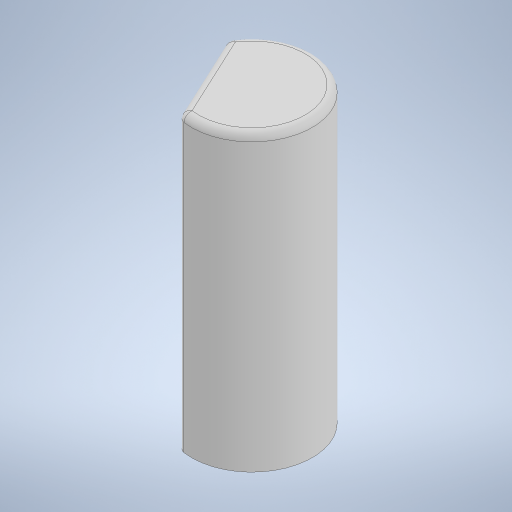
# Autodesk Inventor part: Poti_Verlaengerung
Saved by Autodesk Inventor 2023.1 (Build 271208000, 208)
## iProperties
Created: 2023-12-21
Part Number: Poti_Verlaengerung
Material: Generisch
Document SubType Name: Modeling
Designer: JansenL
Density: 1 g/cm^3
Appearance: Vorgabe
Author: JansenL
Autodesk Inventor part; units mm, degrees
ref_plane "YZ Plane" through (0, 0, 0) normal (1, 0, 0) x (0, 1, 0)
ref_plane "XZ Plane" through (0, 0, 0) normal (0, 1, 0) x (-1, 0, 0)
ref_plane "XY Plane" through (0, 0, 0) normal (0, 0, 1) x (1, 0, 0)
sketch "Sketch1" plane through (0, 0, 0) normal (0, 1, 0) x (-1, 0, 0)
  arc A0 (0.8395, 4.1153) -> (3.6921, -2.0022) centre (0, 0) ccw
  line L0 (0, -7.6704) -> (0, 6.9519) projected
  line L1 (-7.5059, 0) -> (5.9652, 0) projected
  line L2 (3.6921, -2.0022) -> (0.8395, 4.1153)
  dimension "d2" = 8.4
  dimension "d3" = 2.5
  dimension "d4" = 25
  constraints: 2 end point, 2 point on circle, 2 point on line, 1 centre point
  measures "d2" diameter of A0
  measures "d3" distance from line of A0.centre L2
  measures "d4" angle of L0 L2
extrude "Extrusion1" add sketch "Sketch1" along normal blind 20.4
shell "Shell1" thickness 1 removed faces 1 at (-0.173, 0, 1.1178)
fillet "Fillet1" radius 0.5 2 edges at (-2.2658, 20.4, 1.0565) (3.8065, 20.4, -1.775)
fillet "Fillet2" radius 0.5 4 edges at (-3.5246, 20.2564, -1.9963) (-0.7363, 20.2564, 3.9832) (-0.8395, 9.95, 4.1153) (-3.6921, 9.95, -2.0022)
body "Solid1"
